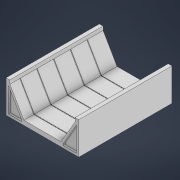
# Autodesk Inventor part: McCrea_Kanal_Walle
Saved by Autodesk Inventor 2022 (Build 260153000, 153)
## iProperties
Created: 2022-02-21
Part Number: McCrea_Kanal_Walle
Material: Generic
Document SubType Name: Modeling
Designer: Lukas
Density: 1 g/cm^3
Appearance: Default
Author: Lukas
Autodesk Inventor part; units mm, degrees
ref_plane "YZ Plane" through (0, 0, 0) normal (1, 0, 0) x (0, 1, 0)
ref_plane "XZ Plane" through (0, 0, 0) normal (0, 1, 0) x (-1, 0, 0)
ref_plane "XY Plane" through (0, 0, 0) normal (0, 0, 1) x (1, 0, 0)
sketch "Sketch1" plane through (0, 0, 0) normal (0, 0, 1) x (1, 0, 0)
  line L0 (0, 0) -> (0, -200)
  line L1 (0, 0) -> (3500, 0)
  line L2 (3500, 0) -> (3500, -200)
  line L3 (1750, 0) -> (1750, -1500)
  line L4 (1750, -1500) -> (750, -1500)
  line L5 (1750, -1500) -> (2750, -1500)
  line L6 (0, -200) -> (750, -1500)
  line L7 (2750, -1500) -> (3500, -200)
  line L8 (0, -200) -> (0, -1500)
  line L9 (0, -1500) -> (750, -1500)
  line L10 (2750, -1500) -> (3500, -1500)
  line L11 (3500, -1500) -> (3500, -200)
  line L12 (0, -1500) -> (3500, -1500)
  line L13 (3500, -1500) -> (3500, -1740.7997)
  line L14 (3500, -1740.7997) -> (0, -1740.7997)
  line L15 (0, -1740.7997) -> (0, -1500)
  line L16 (0, 0) -> (-200, 0)
  line L17 (-200, 0) -> (-200, -1740.7997)
  line L18 (-200, -1740.7997) -> (0, -1740.7997)
  line L19 (0, -1740.7997) -> (0, 0)
  line L20 (3500, 0) -> (3700, 0)
  line L21 (3700, 0) -> (3700, -1740.7997)
  line L22 (3700, -1740.7997) -> (3500, -1740.7997)
  line L23 (3500, -1740.7997) -> (3500, 0)
  dimension "d0" = 200
  dimension "d1" = 3500
  dimension "d2" = 200
  dimension "d3" = 1500
  dimension "d4" = 1000
  dimension "d5" = 1000
  dimension "d6" = 200
  dimension "d7" = 200
  constraints: 48 end point, 6 horizontal, 6 parallel, 5 perpendicular, 4 vertical, 3 point on line, 1 midpoint
  measures "d0" distance of L0.start L0.end
  measures "d1" distance of L0.start L1.end
  measures "d2" distance of L1.end L2.end
  measures "d3" distance of L3.start L3.end
  measures "d4" distance of L3.end L4.end
  measures "d5" distance of L3.end L5.end
  measures "d6" distance of L18.end L17.end
  measures "d7" distance of L21.end L22.end
extrude "Extrusion1" add sketch "Sketch1" against normal blind 5000 contours L0 L8 L15 L18 L17 L16 | L6 L9 L8 | L4 L5 L10 L13 L14 L15 L9 | L20 L21 L22 L13 L11 L2 | L11 L10 L7
sketch "Sketch2" plane through (0, 0, -5000) normal (0, 0, -1) x (-1, 0, 0)
  line L0 (-3700, 0) -> (-3500, 0) projected
  line L1 (-3700, -1740.7997) -> (-3700, 0)
  line L2 (-3700, 0) -> (-3500, 0)
  line L3 (-3500, 0) -> (-3500, -200) projected
  line L4 (-3500, 0) -> (-3500, -200)
  line L5 (-3500, -200) -> (-2750, -1500) projected
  line L6 (-3500, -200) -> (-2750, -1500)
  line L7 (-2750, -1500) -> (-2750, -1740.7997)
  line L8 (-2750, -1740.7997) -> (-3700, -1740.7997)
  line L9 (-3580, -301.4666) -> (-3580, -1620.7997)
  line L10 (-3580, -1620.7997) -> (-2870, -1620.7997)
  line L11 (-2870, -1620.7997) -> (-2870, -1532.1333)
  line L12 (-2870, -1532.1333) -> (-3580, -301.4666)
  line L13 (0, -200) -> (0, 0) projected
  line L14 (0, 0) -> (0, -200)
  line L15 (-750, -1500) -> (0, -200) projected
  line L16 (0, -200) -> (-750, -1500)
  line L17 (-750, -1500) -> (-750, -1740.7997)
  line L18 (200, -1740.7997) -> (200, 0) projected
  line L19 (-750, -1740.7997) -> (200, -1740.7997)
  line L20 (200, -1740.7997) -> (200, 0)
  line L21 (200, 0) -> (0, 0) projected
  line L22 (200, 0) -> (0, 0)
  line L23 (80, -1620.7997) -> (-630, -1620.7997)
  line L24 (-630, -1620.7997) -> (-630, -1532.1333)
  line L25 (-630, -1532.1333) -> (80, -301.4666)
  line L26 (80, -301.4666) -> (80, -1620.7997)
  dimension "d10" = 120
  dimension "d11" = 120
  constraints: 40 end point, 6 collinear, 5 perpendicular, 2 parallel, 1 horizontal, 6 other
  measures "d10" distance between parallel lines of L1 L9
  measures "d11" distance between parallel lines of L19 L23
extrude "Extrusion2" cut sketch "Sketch2" against normal blind 5000 contours L12 L11 L10 L9 | L23 L24 L25 L26
extrude "Extrusion3" add sketch "Sketch2" along normal blind 100 and the other way blind 4900 contours L12 L11 L10 L9 | L23 L24 L25 L26
sketch "Sketch7" plane through (750, -1500, 0) normal (0.8661856, 0.4997225, 0) x (0, 0, -1)
  line L0 (0, 1500.8331) -> (5000, 1500.8331) projected
  line L1 (0, 0) -> (5000, 0) projected
  line L2 (527.4343, 1500.8331) -> (564.3593, 1500.8331)
  line L3 (564.3593, 1500.8331) -> (564.3593, 0)
  line L4 (564.3593, 0) -> (527.4343, 0)
  line L5 (527.4343, 0) -> (527.4343, 1500.8331)
  line L6 (1427.4343, 1500.8331) -> (1464.3593, 1500.8331)
  line L7 (1427.4343, 0) -> (1427.4343, 1500.8331)
  line L8 (1464.3593, 1500.8331) -> (1464.3593, 0)
  line L9 (1464.3593, 0) -> (1427.4343, 0)
  line L10 (2327.4343, 1500.8331) -> (2364.3593, 1500.8331)
  line L11 (2327.4343, 0) -> (2327.4343, 1500.8331)
  line L12 (2364.3593, 1500.8331) -> (2364.3593, 0)
  line L13 (2364.3593, 0) -> (2327.4343, 0)
  line L14 (3227.4343, 1500.8331) -> (3264.3593, 1500.8331)
  line L15 (3227.4343, 0) -> (3227.4343, 1500.8331)
  line L16 (3264.3593, 1500.8331) -> (3264.3593, 0)
  line L17 (3264.3593, 0) -> (3227.4343, 0)
  line L18 (4127.4343, 1500.8331) -> (4164.3593, 1500.8331)
  line L19 (4127.4343, 0) -> (4127.4343, 1500.8331)
  line L20 (4164.3593, 1500.8331) -> (4164.3593, 0)
  line L21 (4164.3593, 0) -> (4127.4343, 0)
  point P0 (0, 1674.0702)
  dimension "d21" = 36.925
  dimension "d24" = 900
  constraints: 40 end point, 2 horizontal, 2 parallel, 2 point on line, 1 perpendicular, 32 other
  measures "d21" distance of L3.end L4.end
  measures "d24" distance of L2.start L6.start
sketch "Sketch8" plane through (750, -1500, 0) normal (0, 1, 0) x (1, 0, 0)
  line L0 (0, 0) -> (0, 5000) projected
  line L1 (0, 527.4032) -> (2000, 527.4032)
  line L2 (2000, 527.4032) -> (2000, 564.3282)
  line L3 (2000, 564.3282) -> (0, 564.3282)
  line L4 (0, 564.3282) -> (0, 527.4032)
  line L5 (0, 1464.3282) -> (0, 1427.4032)
  line L6 (2000, 1464.3282) -> (0, 1464.3282)
  line L7 (0, 1427.4032) -> (2000, 1427.4032)
  line L8 (2000, 1427.4032) -> (2000, 1464.3282)
  line L9 (0, 2364.3282) -> (0, 2327.4032)
  line L10 (2000, 2364.3282) -> (0, 2364.3282)
  line L11 (0, 2327.4032) -> (2000, 2327.4032)
  line L12 (2000, 2327.4032) -> (2000, 2364.3282)
  line L13 (0, 3264.3282) -> (0, 3227.4032)
  line L14 (2000, 3264.3282) -> (0, 3264.3282)
  line L15 (0, 3227.4032) -> (2000, 3227.4032)
  line L16 (2000, 3227.4032) -> (2000, 3264.3282)
  line L17 (0, 4164.3282) -> (0, 4127.4032)
  line L18 (2000, 4164.3282) -> (0, 4164.3282)
  line L19 (0, 4127.4032) -> (2000, 4127.4032)
  line L20 (2000, 4127.4032) -> (2000, 4164.3282)
  point P0 (-750, 0)
  dimension "d29" = 2000
  dimension "d30" = 36.925
  dimension "d33" = 900
  constraints: 40 end point, 2 parallel, 1 horizontal, 1 perpendicular, 1 point on line, 1 vertical, 32 other
  measures "d29" distance of L3.end L2.end
  measures "d30" distance of L2.end L1.end
  measures "d33" distance of L3.end L5.start
sketch "Sketch9" plane through (3500, -200, -5000) normal (-0.8661856, 0.4997225, 0) x (0, 0, 1)
  line L0 (5000, -1500.8331) -> (0, -1500.8331) projected
  line L1 (5000, 0) -> (0, 0) projected
  line L2 (4472.5741, -1500.8331) -> (4435.6491, -1500.8331)
  line L3 (4435.6491, -1500.8331) -> (4435.6491, 0)
  line L4 (4435.6491, 0) -> (4472.5741, 0)
  line L5 (4472.5741, 0) -> (4472.5741, -1500.8331)
  line L6 (3535.6491, 0) -> (3572.5741, 0)
  line L7 (3535.6491, -1500.8331) -> (3535.6491, 0)
  line L8 (3572.5741, 0) -> (3572.5741, -1500.8331)
  line L9 (3572.5741, -1500.8331) -> (3535.6491, -1500.8331)
  line L10 (2635.6491, 0) -> (2672.5741, 0)
  line L11 (2635.6491, -1500.8331) -> (2635.6491, 0)
  line L12 (2672.5741, 0) -> (2672.5741, -1500.8331)
  line L13 (2672.5741, -1500.8331) -> (2635.6491, -1500.8331)
  line L14 (1735.6491, 0) -> (1772.5741, 0)
  line L15 (1735.6491, -1500.8331) -> (1735.6491, 0)
  line L16 (1772.5741, 0) -> (1772.5741, -1500.8331)
  line L17 (1772.5741, -1500.8331) -> (1735.6491, -1500.8331)
  line L18 (835.6491, 0) -> (872.5741, 0)
  line L19 (835.6491, -1500.8331) -> (835.6491, 0)
  line L20 (872.5741, 0) -> (872.5741, -1500.8331)
  line L21 (872.5741, -1500.8331) -> (835.6491, -1500.8331)
  point P0 (5000, -1575.7915)
  point P1 (4472.5741, 0)
  point P2 (3572.5741, -1500.8331)
  point P3 (3572.5741, 0)
  point P4 (3535.6491, 0)
  point P5 (2672.5741, -1500.8331)
  point P6 (2672.5741, 0)
  point P7 (2635.6491, 0)
  point P8 (1772.5741, -1500.8331)
  point P9 (1772.5741, 0)
  point P10 (1735.6491, 0)
  point P11 (872.5741, -1500.8331)
  point P12 (872.5741, 0)
  point P13 (835.6491, 0)
  dimension "d38" = 36.925
  dimension "d41" = 900
  constraints: 40 end point, 2 horizontal, 2 parallel, 2 point on line, 1 perpendicular, 32 other
  measures "d38" distance of L3.end L4.end
  measures "d41" distance of L3.end L6.start
extrude "Extrusion4" cut sketch "Sketch7" against normal blind 10 contours L0 L3 L1 L5 | L0 L8 L1 L7 | L0 L12 L1 L11 | L0 L16 L1 L15 | L0 L20 L1 L19
extrude "Extrusion5" cut sketch "Sketch8" against normal blind 10
extrude "Extrusion6" cut sketch "Sketch9" against normal blind 10 contours L0 L3 L1 L5 | L0 L7 L1 L8 | L0 L11 L1 L12 | L0 L15 L1 L16 | L0 L19 L1 L20
body "Solid1"
